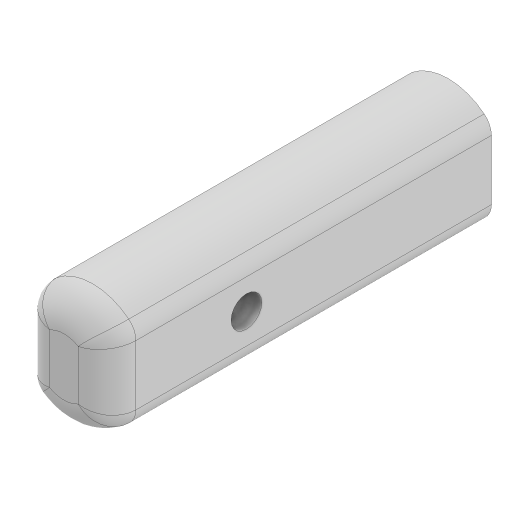
# Autodesk Inventor part: leg
Saved by Autodesk Inventor 2024 (Build 280153000, 153)
## iProperties
Created: 2023-11-07
Part Number: leg
Material: 一般
Document SubType Name: Modeling
Designer: bonju
Density: 1 g/cm^3
Appearance: 既定
Author: bonju
Autodesk Inventor part; units mm, degrees
ref_plane "YZ Plane" through (0, 0, 0) normal (1, 0, 0) x (0, 1, 0)
ref_plane "XZ Plane" through (0, 0, 0) normal (0, 1, 0) x (-1, 0, 0)
ref_plane "XY Plane" through (0, 0, 0) normal (0, 0, 1) x (1, 0, 0)
sketch "スケッチ1" plane through (0, 0, 0) normal (0, 0, 1) x (1, 0, 0)
  line L0 (0, -8.4) -> (0, 8.4) projected
  arc A0 (-4.5, -3.9686) -> (4.5, -3.9686) centre (0, 0) ccw
  arc A1 (4.5, 3.9686) -> (-4.5, 3.9686) centre (0, 0) ccw
  line L1 (-4.5, -3.9686) -> (-4.5, 3.9686)
  line L2 (4.5, -3.9686) -> (4.5, 3.9686)
  line L3 (-3, 3) -> (3, 3)
  line L4 (3, 3) -> (3, -3)
  line L5 (3, -3) -> (-3, -3)
  line L6 (-3, -3) -> (-3, 3)
  line L7 (-3, 3) -> (3, -3) construction
  line L8 (3, 3) -> (-3, -3) construction
  dimension "d22" = 6
  dimension "d23" = 6
  dimension "d24" = 6
  dimension "d25" = 6
  dimension "d26" = 1.5
  constraints: 16 end point, 4 point on circle, 3 parallel, 2 centre point, 2 midpoint, 2 symmetric about line, 1 coincident, 1 horizontal, 1 perpendicular, 1 vertical
  measures "d22" radius of A1
  measures "d23" radius of A0
  measures "d24" distance of L4.end L5.end
  measures "d25" distance of L3.end L4.end
  measures "d26" distance between parallel lines of L6 L1
extrude "押し出し1" add sketch "スケッチ1" along normal blind 40
sketch "スケッチ2" plane through (0, 0, 0) normal (0, 0, -1) x (-1, 0, 0)
  line L0 (3.05, 3.05) -> (-3.05, 3.05)
  line L1 (-3.05, 3.05) -> (-3.05, -3.05)
  line L2 (-3.05, -3.05) -> (3.05, -3.05)
  line L3 (3.05, -3.05) -> (3.05, 3.05)
  line L4 (3.05, 3.05) -> (-3.05, -3.05) construction
  line L5 (-3.05, 3.05) -> (3.05, -3.05) construction
  point P0 (0, 0)
  dimension "d27" = 6.1
  dimension "d28" = 6.1
  constraints: 12 end point, 2 midpoint, 2 parallel, 1 horizontal, 1 perpendicular
  measures "d27" distance of L2.end L1.end
  measures "d28" distance of L1.end L0.end
extrude "押し出し2" cut sketch "スケッチ2" against normal blind 3.1
sketch "スケッチ4" plane through (-4.5, -3.9686, 0) normal (-1, 0, 0) x (0, 0, 1)
  circle A0 centre (25.5, 3.9686) radius 1.6
  line L0 (40, 7.9373) -> (40, 0) projected
  line L1 (0, 3.9686) -> (40, 3.9686) construction
  dimension "d16" = 3.2
  dimension "d17" = 14.5
  constraints: 2 end point, 1 centre point, 1 midpoint, 1 point on line
  measures "d16" diameter of A0
  measures "d17" distance from line of L0 A0.centre
extrude "押し出し4" cut sketch "スケッチ4" along normal through all both and the other way through all
fillet "フィレット1" radius 3 4 edges at (0, -6, 40) (0, 6, 40) (-4.5, 0, 40) (4.5, 0, 40)
fillet "フィレット2" radius 2 8 edges at (3.5186, -3.5785, 39.2193) (4.5, -3.9686, 18.5) (3.5186, 3.5785, 39.2193) (4.5, 3.9686, 18.5) (-3.5186, -3.5785, 39.2193) (-4.5, -3.9686, 18.5) (-3.5186, 3.5785, 39.2193) (-4.5, 3.9686, 18.5)
